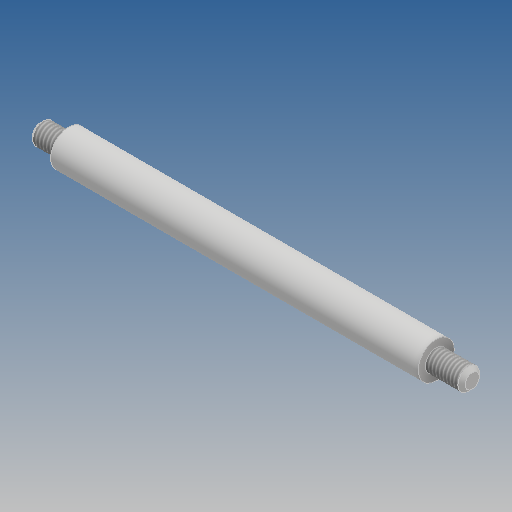
# Autodesk Inventor part: Kolbenstange
Saved by Autodesk Inventor 2018 (Build 220112000, 112)
## iProperties
Created: 2018-10-02
Part Number: Kolbenstange
Material: Generisch
Document SubType Name: Modeling
Designer: M.Knabel
Density: 1 g/cm^3
Appearance: Vorgabe
Mass: 1.06291 g
Surface Area: 9.19027 cm^2
Volume: 1.06291 cm^3
Author: M.Knabel
Autodesk Inventor part; units mm, degrees
ref_plane "YZ Plane" through (0, 0, 0) normal (1, 0, 0) x (0, 1, 0)
ref_plane "XZ Plane" through (0, 0, 0) normal (0, 1, 0) x (-1, 0, 0)
ref_plane "XY Plane" through (0, 0, 0) normal (0, 0, 1) x (1, 0, 0)
sketch "Skizze2" plane through (0, 0, 0) normal (0, 0, 1) x (1, 0, 0)
  line L0 (0, -0.5) -> (0, 3) projected
  line L1 (-12, 0) -> (72, 0) projected
  line L2 (0, 0) -> (4, 0)
  line L3 (4, 1.5) -> (0, 1.5)
  line L4 (0, 1.5) -> (0, 0)
  line L5 (4, 0) -> (55, 0)
  line L6 (55, 1.5) -> (55, 2.5)
  line L7 (55, 2.5) -> (4, 2.5)
  line L8 (4, 2.5) -> (4, 1.5)
  line L9 (55, 0) -> (60, 0)
  line L10 (60, 0) -> (60, 1.5)
  line L11 (60, 1.5) -> (55, 1.5)
  dimension "d0" = 3
  dimension "d1" = 5
  dimension "d2" = 4
  dimension "d3" = 5
  dimension "d4" = 60
  constraints: 20 end point, 4 parallel, 3 horizontal, 2 perpendicular, 2 point on line
  measures "d0" diameter of L3 L1
  measures "d1" diameter of L7 L1
  measures "d2" distance between parallel lines of L8 L0
  measures "d3" distance between parallel lines of L10 L6
  measures "d4" distance between parallel lines of L10 L0
revolve "Umdrehung1" add sketch "Skizze2" angle 360 about axis through (-10, 0, 0) along (1, 0, 0)
thread "Gewinde1" size "M3x0.5" class "6g" standard "ANSI Metric M Profile" full length
thread "Gewinde2" size "M3x0.5" class "6g" standard "ANSI Metric M Profile" full length
chamfer "Fase1" distance 0.5 angle 45 2 edges at (60, -1.5, 0) (0, -1.5, 0)
